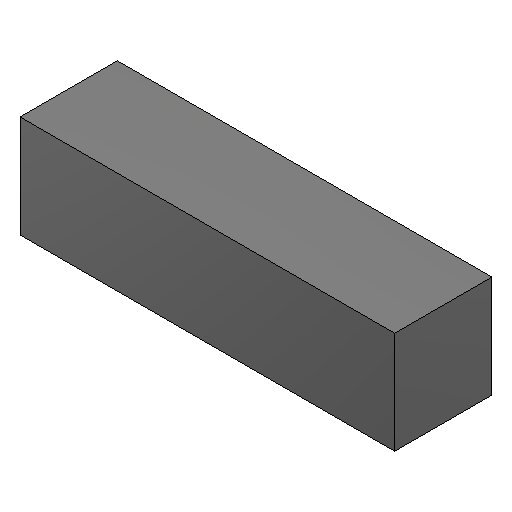
# Autodesk Inventor part: battery-holder
Saved by Autodesk Inventor 2026 (Build 300175050, 175E)
## iProperties
Created: 2025-06-22
Part Number: battery-holder
Material: ABS Plastic
Document SubType Name: Modeling
Designer: queezz
Density: 1.06 g/cm^3
Appearance: Smooth - Black
Author: queezz
Autodesk Inventor part; units mm, degrees
ref_plane "YZ Plane" through (0, 0, 0) normal (1, 0, 0) x (0, 1, 0)
ref_plane "XZ Plane" through (0, 0, 0) normal (0, 1, 0) x (-1, 0, 0)
ref_plane "XY Plane" through (0, 0, 0) normal (0, 0, 1) x (1, 0, 0)
sketch "Sketch1" plane through (0, 0, 0) normal (0, 0, 1) x (1, 0, 0)
  line L0 (-38.5, 10.5) -> (38.5, 10.5)
  line L1 (38.5, 10.5) -> (38.5, -10.5)
  line L2 (38.5, -10.5) -> (-38.5, -10.5)
  line L3 (-38.5, -10.5) -> (-38.5, 10.5)
  point P0 (0, 0)
  point P1 (38.5, 0)
  point P2 (0, 10.5)
  dimension "d0" = 77
  dimension "d1" = 21
  constraints: 8 end point, 2 midpoint, 2 parallel, 1 horizontal, 1 horizontal alignment, 1 perpendicular, 1 vertical alignment
  measures "d0" distance of L0.start L0.end
  measures "d1" distance of L0.end L1.end
extrude "Extrusion1" add sketch "Sketch1" along normal blind 20
body "Solid1"
